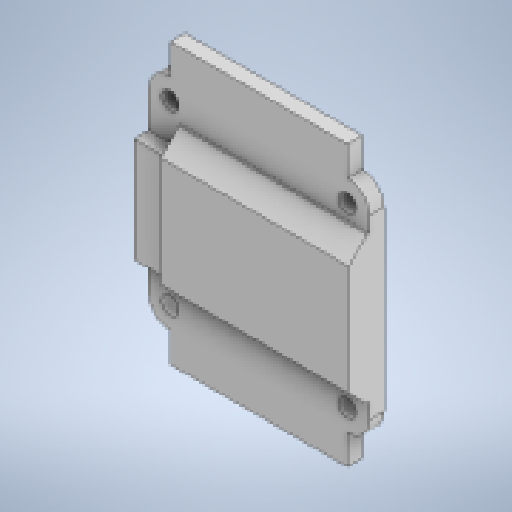
# Autodesk Inventor part: Velox ESC
Saved by Autodesk Inventor 2023 (Build 270158000, 158)
## iProperties
Created: 2022-11-05
Part Number: Velox ESC
Material: Generic
Document SubType Name: Modeling
Designer: mjlangfo
Density: 1 g/cm^3
Appearance: Default
Author: mjlangfo
Autodesk Inventor part; units mm, degrees
ref_plane "YZ Plane" through (0, 0, 0) normal (1, 0, 0) x (0, 1, 0)
ref_plane "XZ Plane" through (0, 0, 0) normal (0, 1, 0) x (-1, 0, 0)
ref_plane "XY Plane" through (0, 0, 0) normal (0, 0, 1) x (1, 0, 0)
sketch "Sketch1" plane through (0, 0, 0) normal (0, 0, 1) x (1, 0, 0)
  arc A0 (15.6734, 13.8392) -> (14.75, 12.1537) centre (16.75, 12.1537) ccw construction
  line L0 (15.6734, 13.8392) -> (18.0766, 15.3743) construction
  arc A1 (18.0766, 15.3743) -> (19, 17.0598) centre (17, 17.0598) ccw construction
  line L1 (19, 17.0598) -> (19, 30.7058) construction
  arc A2 (24.5861, 42.384) -> (19, 30.7058) centre (34, 30.7058) ccw construction
  line L2 (24.5861, 42.384) -> (28.2876, 45.3677) construction
  arc A3 (28.2876, 45.3677) -> (28.7404, 49.5861) centre (26.4048, 47.7034) ccw construction
  line L3 (28.7404, 49.5861) -> (26.2301, 52.7003) construction
  arc A4 (26.2301, 52.7003) -> (22.0117, 53.1532) centre (23.8944, 50.8175) ccw construction
  line L4 (22.0117, 53.1532) -> (11.4653, 44.6517) construction
  arc A5 (2.0515, 41.3299) -> (11.4653, 44.6517) centre (2.0515, 56.3299) ccw construction
  line L5 (2.0515, 41.3299) -> (-2.0515, 41.3299) construction
  arc A6 (-11.4653, 44.6517) -> (-2.0515, 41.3299) centre (-2.0515, 56.3299) ccw construction
  line L6 (-11.4653, 44.6517) -> (-22.0117, 53.1532) construction
  arc A7 (-22.0117, 53.1532) -> (-26.2301, 52.7003) centre (-23.8944, 50.8175) ccw construction
  line L7 (-26.2301, 52.7003) -> (-28.7404, 49.5861) construction
  arc A8 (-28.7404, 49.5861) -> (-28.2876, 45.3677) centre (-26.4048, 47.7034) ccw construction
  line L8 (-28.2876, 45.3677) -> (-24.5861, 42.384) construction
  arc A9 (-19, 30.7058) -> (-24.5861, 42.384) centre (-34, 30.7058) ccw construction
  line L9 (-19, 30.7058) -> (-19, 17.0598) construction
  arc A10 (-19, 17.0598) -> (-18.0766, 15.3743) centre (-17, 17.0598) ccw construction
  line L10 (-18.0766, 15.3743) -> (-15.6734, 13.8392) construction
  arc A11 (-14.75, 12.1537) -> (-15.6734, 13.8392) centre (-16.75, 12.1537) ccw construction
  line L11 (-14.75, 12.1537) -> (-14.75, -5.494) construction
  arc A12 (-15.6734, -7.1795) -> (-14.75, -5.494) centre (-16.75, -5.494) ccw construction
  line L12 (-15.6734, -7.1795) -> (-18.0766, -8.7146) construction
  arc A13 (-18.0766, -8.7146) -> (-19, -10.4001) centre (-17, -10.4001) ccw construction
  line L13 (-19, -10.4001) -> (-19, -30.7058) construction
  arc A14 (-24.5861, -42.384) -> (-19, -30.7058) centre (-34, -30.7058) ccw construction
  line L14 (-24.5861, -42.384) -> (-28.2876, -45.3677) construction
  arc A15 (-28.2876, -45.3677) -> (-28.7404, -49.5861) centre (-26.4048, -47.7034) ccw construction
  line L15 (-28.7404, -49.5861) -> (-26.2301, -52.7003) construction
  arc A16 (-26.2301, -52.7003) -> (-22.0117, -53.1532) centre (-23.8944, -50.8175) ccw construction
  line L16 (-22.0117, -53.1532) -> (-11.4653, -44.6517) construction
  arc A17 (-2.0515, -41.3299) -> (-11.4653, -44.6517) centre (-2.0515, -56.3299) ccw construction
  line L17 (-2.0515, -41.3299) -> (2.0515, -41.3299) construction
  arc A18 (11.4653, -44.6517) -> (2.0515, -41.3299) centre (2.0515, -56.3299) ccw construction
  line L18 (11.4653, -44.6517) -> (22.0117, -53.1532) construction
  arc A19 (22.0117, -53.1532) -> (26.2301, -52.7003) centre (23.8944, -50.8175) ccw construction
  line L19 (26.2301, -52.7003) -> (28.7404, -49.5861) construction
  arc A20 (28.7404, -49.5861) -> (28.2876, -45.3677) centre (26.4048, -47.7034) ccw construction
  line L20 (28.2876, -45.3677) -> (24.5861, -42.384) construction
  arc A21 (19, -30.7058) -> (24.5861, -42.384) centre (34, -30.7058) ccw construction
  line L21 (19, -30.7058) -> (19, -10.4001) construction
  arc A22 (19, -10.4001) -> (18.0766, -8.7146) centre (17, -10.4001) ccw construction
  line L22 (18.0766, -8.7146) -> (15.6734, -7.1795) construction
  arc A23 (14.75, -5.494) -> (15.6734, -7.1795) centre (16.75, -5.494) ccw construction
  line L23 (14.75, -5.494) -> (14.75, 12.1537) construction
  spline S0 degree 3 poles (8.2673, 8.7575) (8.2937, 7.6146) (8.3178, 6.4713) (8.3615, 4.1764) (8.3811, 3.024) (8.3985, 1.872) knots 0 0 0 0 0.342955 0.342955 0.688597 0.688597 0.688597 0.688597 construction
  arc A24 (7.2587, 0.991) -> (8.3985, 1.872) centre (7.4986, 1.8584) ccw construction
  line L24 (7.2587, 0.991) -> (3.6122, 1.9996) construction
  arc A25 (3.0306, 3.4932) -> (3.6122, 1.9996) centre (3.8788, 2.9634) ccw construction
  line L25 (3.0306, 3.4932) -> (6.6042, 9.2136) construction
  arc A26 (8.2673, 8.7575) -> (6.6042, 9.2136) centre (7.3675, 8.7367) ccw construction
  line L26 (-3.336, -2.3124) -> (-0.2664, -1.464) construction
  arc A27 (0.2664, -1.464) -> (-0.2664, -1.464) centre (0, -2.4278) ccw construction
  line L27 (0.2664, -1.464) -> (3.336, -2.3124) construction
  arc A28 (3.9177, -3.8061) -> (3.336, -2.3124) centre (3.0696, -3.2763) ccw construction
  line L28 (3.9177, -3.8061) -> (0.8481, -8.7198) construction
  arc A29 (-0.8481, -8.7198) -> (0.8481, -8.7198) centre (0, -8.19) ccw construction
  line L29 (-0.8481, -8.7198) -> (-3.9177, -3.8061) construction
  arc A30 (-3.336, -2.3124) -> (-3.9177, -3.8061) centre (-3.0696, -3.2763) ccw construction
  line L30 (6.2794, 18.6976) -> (1.9507, 19.9359) construction
  arc A31 (1.3777, 21.4271) -> (1.9507, 19.9359) centre (2.2258, 20.8973) ccw construction
  line L31 (1.3777, 21.4271) -> (4.6803, 26.7137) construction
  arc A32 (6.5163, 26.3393) -> (4.6803, 26.7137) centre (5.5284, 26.1839) ccw construction
  line L32 (6.5163, 26.3393) -> (7.5423, 19.8143) construction
  arc A33 (6.2794, 18.6976) -> (7.5423, 19.8143) centre (6.5544, 19.659) ccw construction
  line L33 (0.275, 16.6432) -> (4.3044, 15.4905) construction
  arc A34 (4.8775, 13.9992) -> (4.3044, 15.4905) centre (4.0294, 14.529) ccw construction
  line L34 (4.8775, 13.9992) -> (0.8481, 7.5492) construction
  arc A35 (-0.8481, 7.5492) -> (0.8481, 7.5492) centre (0, 8.0791) ccw construction
  line L35 (-0.8481, 7.5492) -> (-4.8775, 13.9992) construction
  arc A36 (-4.3044, 15.4905) -> (-4.8775, 13.9992) centre (-4.0294, 14.529) ccw construction
  line L36 (-4.3044, 15.4905) -> (-0.275, 16.6432) construction
  arc A37 (0.275, 16.6432) -> (-0.275, 16.6432) centre (0, 15.6817) ccw construction
  spline S1 degree 3 poles (-8.3985, 1.872) (-8.3811, 3.024) (-8.3615, 4.1764) (-8.3178, 6.4713) (-8.2937, 7.6146) (-8.2673, 8.7575) knots 0 0 0 0 0.345643 0.345643 0.688601 0.688601 0.688601 0.688601 construction
  arc A38 (-6.6042, 9.2136) -> (-8.2673, 8.7575) centre (-7.3675, 8.7367) ccw construction
  line L37 (-6.6042, 9.2136) -> (-3.0306, 3.4932) construction
  arc A39 (-3.6122, 1.9996) -> (-3.0306, 3.4932) centre (-3.8788, 2.9634) ccw construction
  line L38 (-3.6122, 1.9996) -> (-7.2587, 0.991) construction
  arc A40 (-8.3985, 1.872) -> (-7.2587, 0.991) centre (-7.4986, 1.8584) ccw construction
  line L39 (-4.6803, 26.7137) -> (-1.3777, 21.4271) construction
  arc A41 (-1.9507, 19.9359) -> (-1.3777, 21.4271) centre (-2.2258, 20.8973) ccw construction
  line L40 (-1.9507, 19.9359) -> (-6.2794, 18.6976) construction
  arc A42 (-7.5423, 19.8143) -> (-6.2794, 18.6976) centre (-6.5544, 19.659) ccw construction
  line L41 (-7.5423, 19.8143) -> (-6.5163, 26.3393) construction
  arc A43 (-4.6803, 26.7137) -> (-6.5163, 26.3393) centre (-5.5284, 26.1839) ccw construction
  circle A44 centre (-23.5925, -48.0053) radius 1.475 construction
  arc A45 (3, -16.1701) -> (-3, -16.1701) centre (0, -16.1701) ccw construction
  line L42 (3, -16.1701) -> (3, -28.3299) construction
  arc A46 (-3, -28.3299) -> (3, -28.3299) centre (0, -28.3299) ccw construction
  line L43 (-3, -28.3299) -> (-3, -16.1701) construction
  circle A47 centre (-23.5925, 48.0053) radius 1.475 construction
  circle A48 centre (-10, 13.3299) radius 1.475 construction
  circle A49 centre (-10, -6.6701) radius 1.475 construction
  circle A50 centre (-15.25, -11.9201) radius 1.5 projected
  circle A51 centre (-14.25, -40.4742) radius 1.475 construction
  circle A52 centre (23.5925, -48.0053) radius 1.475 construction
  circle A53 centre (15.25, -11.9201) radius 1.5 projected
  circle A54 centre (14.25, 40.4742) radius 1.475 construction
  circle A55 centre (10, 13.3299) radius 1.475 construction
  circle A56 centre (14.25, -40.4742) radius 1.475 construction
  circle A57 centre (15.25, 18.5799) radius 1.5 projected
  circle A58 centre (-15.25, 18.5799) radius 1.5 projected
  circle A59 centre (10, -6.6701) radius 1.475 construction
  circle A60 centre (-14.25, 40.4742) radius 1.475 construction
  circle A61 centre (23.5925, 48.0053) radius 1.475 construction
  line L44 (19, 22.3299) -> (15.25, 22.3299) construction
  line L45 (-19, 22.3299) -> (-19, 18.5799) construction
  line L46 (-19, -15.6701) -> (-15.25, -15.6701) construction
  line L47 (19, -15.6701) -> (19, -11.9201) construction
  arc A62 (19, 18.5799) -> (15.25, 22.3299) centre (15.25, 18.5799) ccw
  arc A63 (-15.25, 22.3299) -> (-19, 18.5799) centre (-15.25, 18.5799) ccw
  arc A64 (15.25, -15.6701) -> (19, -11.9201) centre (15.25, -11.9201) ccw
  arc A65 (-19, -11.9201) -> (-15.25, -15.6701) centre (-15.25, -11.9201) ccw
  arc A66 (-19, 18.5799) -> (-15.25, 22.3299) centre (-15.25, 18.5799) ccw construction
  arc A67 (15.25, 22.3299) -> (19, 18.5799) centre (15.25, 18.5799) ccw construction
  arc A68 (19, -11.9201) -> (15.25, -15.6701) centre (15.25, -11.9201) ccw construction
  arc A69 (-15.25, -15.6701) -> (-19, -11.9201) centre (-15.25, -11.9201) ccw construction
  line L48 (19, 18.5799) -> (19, 22.3299) construction
  line L49 (15.25, 22.3299) -> (-15.25, 22.3299)
  line L50 (-15.25, 22.3299) -> (-19, 22.3299) construction
  line L51 (-19, 18.5799) -> (-19, -11.9201)
  line L52 (-19, -11.9201) -> (-19, -15.6701) construction
  line L53 (-15.25, -15.6701) -> (15.25, -15.6701)
  line L54 (15.25, -15.6701) -> (19, -15.6701) construction
  line L55 (19, -11.9201) -> (19, 18.5799)
  point P0 (0, 0)
  dimension "d0" = 3.75
  dimension "d1" = 3.75
  dimension "d2" = 3.75
  constraints: 24 end point, 18 parallel, 16 point on circle, 12 tangent, 9 perpendicular, 8 centre point, 5 point on line, 4 coincident, 3 horizontal
  measures "d0" distance from line of L9 A58.centre
  measures "d1" distance from line of A58.centre L44
  measures "d2" distance from line of A50.centre L46
extrude "Extrusion1" add sketch "Sketch1" along normal blind 2.54
sketch "Sketch2" plane through (0, 0, 2.54) normal (0, 0, 1) x (1, 0, 0)
  line L0 (-13.92, 12.3346) -> (-19, 12.3346)
  line L1 (-19, 12.3346) -> (-19, -5.6749)
  line L2 (-19, -5.6749) -> (-13.92, -5.6749)
  line L3 (-13.92, -5.6749) -> (-13.92, 12.3346)
  line L4 (15.25, 22.3299) -> (-15.25, 22.3299) construction
  line L5 (-15.25, -15.6701) -> (15.25, -15.6701) construction
  line L6 (-19, 18.5799) -> (-19, -11.9201) construction
  point P0 (0, 0)
  dimension "d5" = 9.9953
  dimension "d6" = 9.9953
  dimension "d7" = 5.08
  constraints: 8 end point, 2 parallel, 1 horizontal, 1 perpendicular, 1 point on line
  measures "d5" distance from line of L4.end L0
  measures "d6" distance from line of L5.start L2
  measures "d7" distance of L1.end L2.end
extrude "Extrusion2" add sketch "Sketch2" along normal blind 2.54
sketch "Sketch3" plane through (0, 0, 2.54) normal (0, 0, 1) x (1, 0, 0)
  line L0 (19, -11.9201) -> (19, 18.5799) projected
  line L1 (19, 15.9799) -> (-13.3786, 15.9799)
  line L2 (-13.3786, 15.9799) -> (-13.3786, -9.3201)
  line L3 (-13.3786, -9.3201) -> (19, -9.3201)
  line L4 (19, -9.3201) -> (19, 15.9799)
  line L5 (15.25, 22.3299) -> (-15.25, 22.3299) projected
  line L6 (-15.25, -15.6701) -> (15.25, -15.6701) projected
  point P0 (0, 0)
  dimension "d10" = 6.35
  dimension "d11" = 6.35
  constraints: 8 end point, 2 parallel, 1 horizontal, 1 perpendicular, 1 point on line
  measures "d10" distance from line of L5.start L1
  measures "d11" distance from line of L6.end L3
extrude "Extrusion3" add sketch "Sketch3" along normal blind 3.556
chamfer "Chamfer1" distance 3.175 angle 45 1 edges at (2.8107, 15.9799, 6.096)
chamfer "Chamfer2" distance 3.175 angle 45 1 edges at (2.8107, -9.3201, 6.096)
sketch "Sketch4" plane through (-15.25, 22.3299, 0) normal (0, 1, 0) x (1, 0, 0)
  line L0 (30.5, 0) -> (0, 0) projected
  line L1 (0, 0) -> (0, -2.54) projected
  line L2 (30.5, -2.54) -> (0, -2.54) projected
  line L3 (30.5, 0) -> (30.5, -2.54) projected
  point P0 (15.25, 0)
extrude "Extrusion4" add sketch "Sketch4" along normal blind 5.08
sketch "Sketch5" plane through (-15.25, -15.6701, 0) normal (0, -1, 0) x (1, 0, 0)
  line L0 (0, 0) -> (30.5, 0) projected
  line L1 (30.5, 0) -> (30.5, 2.54) projected
  line L2 (0, 2.54) -> (30.5, 2.54) projected
  line L3 (0, 0) -> (0, 2.54) projected
  point P0 (15.25, 0)
extrude "Extrusion5" add sketch "Sketch5" along normal blind 5.08
equation "\"d1\" = d0"
equation "\"d2\" = d0"
equation "\"d6\" = d5"
equation "\"d11\" = d10"
body "Solid1"
